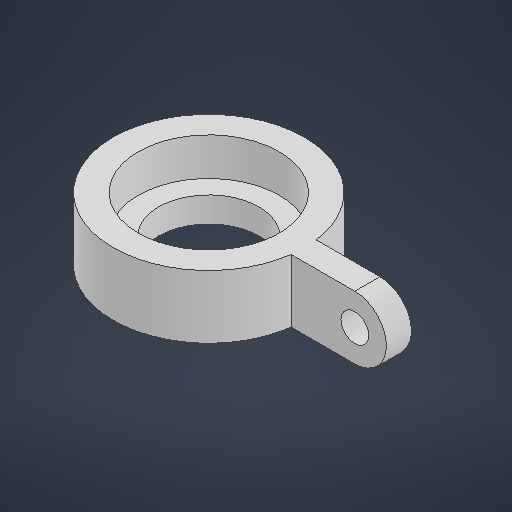
# Autodesk Inventor part: Bearing Grip
Saved by Autodesk Inventor 2025.1 (Build 291241000, 241)
## iProperties
Created: 2025-03-13
Part Number: Bearing Grip
Material: Generic
Document SubType Name: Modeling
Designer: jerem
Density: 1 g/cm^3
Appearance: Default
Author: jerem
## iProperties of the stored document Bearing Grip_3DPrint.ipt
Created: 2025-03-13
Part Number: Bearing Grip_3DPrint
Material: Generic
Document SubType Name: Modeling
Designer: jerem
Density: 1 g/cm^3
Appearance: Default
Author: jerem
Autodesk Inventor part; units mm, degrees
ref_plane "YZ Plane" through (0, 0, 0) normal (1, 0, 0) x (0, 1, 0)
ref_plane "XZ Plane" through (0, 0, 0) normal (0, 1, 0) x (-1, 0, 0)
ref_plane "XY Plane" through (0, 0, 0) normal (0, 0, 1) x (1, 0, 0)
sketch "Sketch1" plane through (0, 0, 0) normal (0, 1, 0) x (-1, 0, 0)
  circle A0 centre (0, 0) radius 4
  circle A1 centre (0, 0) radius 5.6
  circle A2 centre (0, 0) radius 7.6
  dimension "d0" = 8
  dimension "d1" = 11.2
  dimension "d14" = 2
  constraints: 3 centre point, 3 coincident
  measures "d0" diameter of A0
  measures "d1" diameter of A1
  measures "d14" radial gap between concentric circles of A2 A1
extrude "Extrusion1" add sketch "Sketch1" against normal blind 2 contours A1 | A2
extrude "Extrusion2" add sketch "Sketch1" along normal blind 3 contours A2
sketch "Sketch2" plane through (0, 0, 0) normal (0, 0, 1) x (1, 0, 0)
  line L0 (7.6, 3) -> (7.6, -2) projected
  line L1 (7.6, 3) -> (12.6, 3)
  line L2 (7.6, -2) -> (12.6, -2)
  line L3 (7.6, 0.5) -> (12.6, 0.5) construction
  circle A0 centre (12.6, 0.5) radius 2.5
  circle A1 centre (12.6, 0.5) radius 1.1
  line L4 (7.6, 3) -> (6.6, 3)
  line L5 (6.6, 3) -> (6.6, -2)
  line L6 (6.6, -2) -> (7.6, -2)
  point P0 (0, 0)
  dimension "d7" = 2.2
  dimension "d8" = 5
  dimension "d11" = 1
  dimension "d15" = 5
  constraints: 12 end point, 2 centre point, 2 coincident, 2 horizontal, 2 perpendicular, 2 point on circle, 2 tangent, 1 midpoint
  measures "d7" diameter of A1
  measures "d8" diameter of A0
  measures "d11" distance between parallel lines of L0 L5
  measures "d15" distance of L3.start L3.end
extrude "Extrusion3" add sketch "Sketch2" along normal mid plane 2
body "Solid1"
